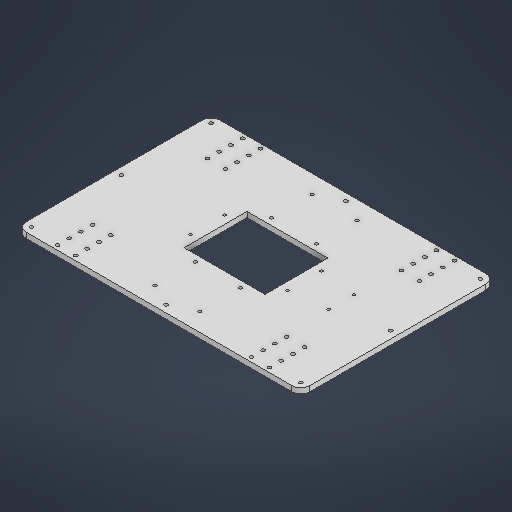
# Autodesk Inventor part: power layer
Saved by Autodesk Inventor 2026.1 (Build 301233000, 233)
## iProperties
Created: 2026-03-06
Part Number: power layer
Material: Generic
Document SubType Name: Modeling
Designer: momen
Density: 1 g/cm^3
Appearance: Default
Author: momen
Autodesk Inventor part; units mm, degrees
ref_plane "YZ Plane" through (0, 0, 0) normal (1, 0, 0) x (0, 1, 0)
ref_plane "XZ Plane" through (0, 0, 0) normal (0, 1, 0) x (-1, 0, 0)
ref_plane "XY Plane" through (0, 0, 0) normal (0, 0, 1) x (1, 0, 0)
sketch "Sketch1" plane through (0, 0, 0) normal (0, 1, 0) x (-1, 0, 0)
  line L0 (-158, 108) -> (158, 108)
  line L1 (158, 108) -> (158, -108)
  line L2 (158, -108) -> (-158, -108)
  line L3 (-158, -108) -> (-158, 108)
  line L4 (-158, 108) -> (158, -108) construction
  line L5 (158, 108) -> (-158, -108) construction
  line L6 (-150, 100) -> (150, 100)
  line L7 (150, 100) -> (150, -100)
  line L8 (150, -100) -> (-150, -100)
  line L9 (-150, -100) -> (-150, 100)
  line L10 (-150, 100) -> (150, -100) construction
  line L11 (150, 100) -> (-150, -100) construction
  circle A0 centre (150, 0) radius 2
  circle A1 centre (150, -100) radius 2
  circle A2 centre (150, 100) radius 2
  circle A3 centre (0, 100) radius 2
  circle A4 centre (0, -100) radius 2
  circle A5 centre (-150, -100) radius 2
  circle A6 centre (-150, 0) radius 2
  circle A7 centre (-150, 100) radius 2
  point P0 (0, 0)
  dimension "d0" = 316
  dimension "d1" = 216
  dimension "d2" = 300
  dimension "d3" = 200
  dimension "d4" = 4
  dimension "d5" = 4
  dimension "d6" = 4
  dimension "d7" = 4
  dimension "d8" = 4
  dimension "d9" = 4
  dimension "d10" = 4
  dimension "d11" = 4
  constraints: 24 end point, 9 coincident, 8 centre point, 8 midpoint, 4 parallel, 2 horizontal, 2 perpendicular
  measures "d0" distance of L1.end L2.end
  measures "d1" distance of L0.end L1.end
  measures "d2" distance of L7.end L8.end
  measures "d3" distance of L6.end L7.end
  measures "d4" diameter of A0
  measures "d5" diameter of A1
  measures "d6" diameter of A2
  measures "d7" diameter of A3
  measures "d8" diameter of A4
  measures "d9" diameter of A5
  measures "d10" diameter of A6
  measures "d11" diameter of A7
extrude "Extrusion1" add sketch "Sketch1" along normal blind 6 contours L0 L1 L2 L3 | L6 A3 A2 L7 A0 A1 L8 A4 A5 L9 A6 A7
sketch "Sketch2" plane through (0, 6, 0) normal (0, 1, 0) x (1, 0, 0)
  line L0 (158, 108) -> (20.8385, 108)
  line L1 (158, 108) -> (108, 108)
  line L2 (108, 108) -> (108, 103)
  line L3 (108, 103) -> (158, 103)
  line L4 (158, 103) -> (158, 108)
  line L5 (98, 64) -> (98, 77)
  line L6 (98, 77) -> (118, 77)
  line L7 (118, 77) -> (118, 64)
  line L8 (118, 64) -> (98, 64)
  line L9 (98, 77) -> (98, 90)
  line L10 (98, 90) -> (118, 90)
  line L11 (118, 90) -> (118, 77)
  line L12 (118, 77) -> (98, 77)
  line L13 (98, 90) -> (98, 103)
  line L14 (98, 103) -> (118, 103)
  line L15 (118, 103) -> (118, 90)
  line L16 (118, 90) -> (98, 90)
  circle A0 centre (118, 103) radius 2
  circle A1 centre (118, 90) radius 2
  circle A2 centre (118, 77) radius 2
  circle A3 centre (118, 64) radius 2
  circle A4 centre (98, 64) radius 2
  circle A5 centre (98, 77) radius 2
  circle A6 centre (98, 90) radius 2
  circle A7 centre (98, 103) radius 2
  line L17 (-158, 108) -> (-108, 108)
  line L18 (-108, 108) -> (-108, 103)
  line L19 (-108, 103) -> (-158, 103)
  line L20 (-98, 64) -> (-98, 77)
  line L21 (-118, 90) -> (-118, 77)
  line L22 (-98, 77) -> (-98, 90)
  line L23 (-98, 77) -> (-118, 77)
  line L24 (-118, 77) -> (-98, 77)
  circle A8 centre (-118, 77) radius 2
  circle A9 centre (-98, 77) radius 2
  line L25 (-118, 77) -> (-118, 64)
  circle A10 centre (-118, 64) radius 2
  circle A11 centre (-98, 64) radius 2
  line L26 (-118, 64) -> (-98, 64)
  line L27 (-98, 90) -> (-118, 90)
  line L28 (-118, 90) -> (-98, 90)
  circle A12 centre (-118, 90) radius 2
  circle A13 centre (-98, 90) radius 2
  line L29 (-98, 90) -> (-98, 103)
  line L30 (-98, 103) -> (-118, 103)
  circle A14 centre (-98, 103) radius 2
  line L31 (-118, 103) -> (-118, 90)
  circle A15 centre (-118, 103) radius 2
  line L32 (158, -108) -> (108, -108)
  line L33 (108, -108) -> (108, -103)
  line L34 (108, -103) -> (158, -103)
  line L35 (98, -64) -> (98, -77)
  line L36 (118, -90) -> (118, -77)
  line L37 (98, -77) -> (98, -90)
  line L38 (98, -77) -> (118, -77)
  line L39 (118, -77) -> (98, -77)
  circle A16 centre (118, -77) radius 2
  circle A17 centre (98, -77) radius 2
  line L40 (118, -77) -> (118, -64)
  circle A18 centre (118, -64) radius 2
  circle A19 centre (98, -64) radius 2
  line L41 (118, -64) -> (98, -64)
  line L42 (98, -90) -> (118, -90)
  line L43 (118, -90) -> (98, -90)
  circle A20 centre (118, -90) radius 2
  circle A21 centre (98, -90) radius 2
  line L44 (98, -90) -> (98, -103)
  line L45 (98, -103) -> (118, -103)
  circle A22 centre (98, -103) radius 2
  line L46 (118, -103) -> (118, -90)
  circle A23 centre (118, -103) radius 2
  line L47 (-118, -90) -> (-118, -77)
  circle A24 centre (-118, -77) radius 2
  line L48 (-118, -77) -> (-118, -64)
  line L49 (-118, -77) -> (-98, -77)
  line L50 (-98, -77) -> (-118, -77)
  line L51 (-98, -77) -> (-98, -90)
  circle A25 centre (-118, -64) radius 2
  circle A26 centre (-98, -77) radius 2
  line L52 (-98, -64) -> (-98, -77)
  line L53 (-118, -64) -> (-98, -64)
  circle A27 centre (-98, -64) radius 2
  line L54 (-108, -103) -> (-158, -103)
  line L55 (-108, -108) -> (-108, -103)
  circle A28 centre (-98, -90) radius 2
  line L56 (-118, -90) -> (-98, -90)
  line L57 (-98, -90) -> (-118, -90)
  circle A29 centre (-118, -90) radius 2
  line L58 (-98, -90) -> (-98, -103)
  circle A30 centre (-98, -103) radius 2
  line L59 (-98, -103) -> (-118, -103)
  line L60 (-118, -103) -> (-118, -90)
  circle A31 centre (-118, -103) radius 2
  line L61 (45, -35) -> (-45, -35)
  line L62 (-45, -35) -> (-45, 35)
  line L63 (-45, 35) -> (45, 35)
  line L64 (45, 35) -> (45, -35)
  line L65 (45, -35) -> (-45, 35) construction
  line L66 (-45, -35) -> (45, 35) construction
  point P0 (0, 0)
  point P1 (-158, -108)
  dimension "d27" = 50
  dimension "d28" = 5
  dimension "d29" = 13
  dimension "d30" = 20
  dimension "d31" = 13
  dimension "d32" = 20
  dimension "d33" = 13
  dimension "d34" = 4
  dimension "d35" = 4
  dimension "d36" = 4
  dimension "d37" = 4
  dimension "d38" = 4
  dimension "d39" = 4
  dimension "d40" = 4
  dimension "d41" = 4
  dimension "d42" = 90
  dimension "d43" = 70
  constraints: 134 end point, 32 centre point, 32 coincident, 10 parallel, 5 perpendicular, 4 point on line, 3 midpoint, 2 horizontal
  measures "d27" distance of L3.end L2.end
  measures "d28" distance of L2.end L1.end
  measures "d29" distance of L6.end L7.end
  measures "d30" distance of L5.end L6.end
  measures "d31" distance of L11.start L11.end
  measures "d32" distance of L9.end L11.start
  measures "d33" distance of L14.end L16.start
  measures "d34" diameter of A0
  measures "d35" diameter of A1
  measures "d36" diameter of A2
  measures "d37" diameter of A3
  measures "d38" diameter of A4
  measures "d39" diameter of A5
  measures "d40" diameter of A6
  measures "d41" diameter of A7
  measures "d42" distance of L62.end L63.end
  measures "d43" distance of L61.end L62.end
extrude "Extrusion2" cut sketch "Sketch2" against normal blind 6 contours A0 L15 L3 | L3 A0 | L3 L15 A0 | A7 L13 L14 | L14 L13 A7 | A1 L11 L15 | L15 L10 A1 | A6 L10 L13 | L13 L9 A6 | L11 A1 L10 | L10 A6 L9 | A5 L6 L9 | L9 L5 A5 | A2 L7 L11 | L11 L6 A2 | L6 A5 L5 | L7 A2 L6 | A4 L8 L5 | L5 L8 A4 | A3 L8 L7 | L7 L8 A3 | A15 L31 L19 | L19 A15 | A14 L29 L30 | L30 L29 A14 | L31 A15 L19 | L31 L21 A12 | A12 L27 L31 | L29 L27 A13 | A13 L22 L29 | A12 L21 L27 | L27 L22 A13 | A8 L23 L21 | L21 L25 A8 | L23 A8 L25 | A9 L20 L22 | L22 L23 A9 | L23 L20 A9 | A10 L26 L25 | L25 L26 A10 | A11 L26 L20 | L20 L26 A11 | L46 A23 L34 | L34 A23 | L34 A23 L46 | L46 L36 A20 | A20 L42 L46 | A22 L44 L45 | L45 L44 A22 | A20 L36 L42 | A21 L44 L42 | L42 L37 A21 | A21 L37 L44 | A16 L38 L36 | L36 L40 A16 | A17 L35 L37 | L37 L38 A17 | L38 A16 L40 | L35 A17 L38 | A19 L41 L35 | L35 L41 A19 | A18 L41 L40 | L40 L41 A18 | L60 A29 L47 | L47 A29 L56 | L56 A29 L60 | A24 L48 L47 | L47 L49 A24 | L56 L58 A28 | A28 L51 L56 | A31 L54 L60 | L60 L54 A31 | L48 A24 L49 | A28 L58 L51 | L54 A31 | A25 L53 L48 | L48 L53 A25 | A26 L52 L49 | L49 L51 A26 | L51 L52 A26 | A30 L59 L58 | L58 L59 A30 | A27 L52 L53 | L53 L52 A27 | L61 L62 L63 L64
fillet "Fillet1" radius 10 5 edges at (-158, 3, 108) (158, 3, 108) (158, 3, -108) (-158, 3, -108) (-148, 0, -100)
sketch "Sketch3" plane through (0, 6, 0) normal (0, 1, 0) x (1, 0, 0)
  line L0 (-45, 35) -> (-45, -35) projected
  line L1 (-158, 92.2115) -> (-158, -98) projected
  line L2 (25.05, -42.45) -> (-25.05, -42.45)
  line L3 (-25.05, -87.55) -> (25.05, -87.55)
  line L4 (158, -98) -> (158, 98) projected
  line L5 (45, -35) -> (45, 35) projected
  line L6 (25.05, 87.55) -> (-25.05, 87.55)
  line L7 (-25.05, 42.45) -> (25.05, 42.45)
  circle A0 centre (-25.05, -42.45) radius 1.75
  circle A1 centre (-25.05, -87.55) radius 1.75
  circle A2 centre (25.05, -42.45) radius 1.75
  circle A3 centre (25.05, -87.55) radius 1.75
  circle A4 centre (25.05, 87.55) radius 1.75
  circle A5 centre (25.05, 42.45) radius 1.75
  circle A6 centre (-25.05, 42.45) radius 1.75
  circle A7 centre (-25.05, 87.55) radius 1.75
  line L8 (-25.05, 87.55) -> (25.05, 42.45)
  circle A8 centre (0, 100) radius 2 projected
  line L9 (0, 100) -> (0, 35)
  line L10 (-45, 35) -> (45, 35) projected
  line L11 (45, -35) -> (-45, -35) projected
  circle A9 centre (0, -100) radius 2 projected
  line L12 (0, -35) -> (0, -100)
  line L13 (-25.05, -42.45) -> (25.05, -87.55)
  line L14 (0, 42.45) -> (0, 39.95)
  line L15 (0, -42.45) -> (0, -39.95)
  line L16 (45, 35) -> (45, -35) projected
  line L17 (45, 35) -> (45, 54)
  line L18 (45, 54) -> (54, 54)
  point P0 (0, 0)
  point P1 (0, 67.5)
  point P2 (0, 65)
  point P3 (0, -65)
  point P4 (0, -67.5)
  dimension "d53" = 3.5
  dimension "d54" = 3.5
  dimension "d55" = 3.5
  dimension "d56" = 3.5
  dimension "d58" = 3.5
  dimension "d59" = 3.5
  dimension "d60" = 3.5
  dimension "d63" = 2.5
  dimension "d64" = 2.5
  dimension "d65" = 19
  dimension "d66" = 9
  constraints: 24 end point, 10 coincident, 8 centre point, 8 midpoint, 5 point on line, 2 parallel, 1 perpendicular, 1 vertical
  measures "d53" diameter of A0
  measures "d54" diameter of A1
  measures "d55" diameter of A2
  measures "d56" diameter of A3
  measures "d58" diameter of A5
  measures "d59" diameter of A6
  measures "d60" diameter of A7
  measures "d63" distance of L14.start L14.end
  measures "d64" distance of L15.start L15.end
  measures "d65" distance of L5.end L17.end
  measures "d66" distance of L17.end L18.end
extrude "Extrusion3" cut sketch "Sketch3" against normal blind 6 contours A0 L13 L2 | L2 L13 A0 | L13 L3 A3 | A3 L3 L13 | A7 L8 L6 | L6 L8 A7 | L8 L7 A5 | A5 L7 L8 | A1 | A2 | A4 | A6
sketch "Sketch4" plane through (0, 0, 0) normal (0, -1, 0) x (1, 0, 0)
  line L0 (-158, 108) -> (158, -108) construction
  circle A0 centre (54, -19) radius 1.5 projected
  circle A1 centre (54, 19) radius 1.5 projected
  circle A2 centre (-54, 19) radius 1.5 projected
  circle A3 centre (-54, -19) radius 1.5 projected
  point P0 (0, 0)
extrude "Extrusion4" cut sketch "Sketch4" against normal blind 10
sketch "Sketch6" plane through (0, 6, 0) normal (0, 1, 0) x (1, 0, 0)
  circle A0 centre (94.95, -14) radius 1.55 projected
  circle A1 centre (94.95, 14) radius 1.55 projected
  circle A2 centre (94.95, -14) radius 1.55
  circle A3 centre (94.95, 14) radius 1.55
  point P0 (0, 0)
  constraints: 2 centre point, 2 coincident, 2 concentric
extrude "Extrusion6" cut sketch "Sketch6" against normal through all
body "Solid1"
